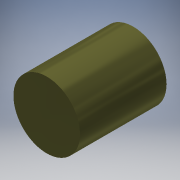
# Autodesk Inventor part: Pin
Saved by Autodesk Inventor 2019 Beta2 (Build 230110000, 110) ContinuousBuild 0
## iProperties
Created: 2014-03-04
Part Number: Pin
Material: Titanium
Document SubType Name: Modeling
Designer: John
Density: 4.51 g/cm^3
Appearance: Titanium
Mass: 1.17905 g
Surface Area: 2.28018 cm^2
Volume: 0.261429 cm^3
Author: John
Autodesk Inventor part; units mm, degrees
ref_plane "YZ Plane" through (0, 0, 0) normal (1, 0, 0) x (0, 1, 0)
ref_plane "XZ Plane" through (0, 0, 0) normal (0, 1, 0) x (-1, 0, 0)
ref_plane "XY Plane" through (0, 0, 0) normal (0, 0, 1) x (1, 0, 0)
sketch "Sketch1" plane through (0, 0, 0) normal (0, 0, 1) x (1, 0, 0)
  circle A0 centre (0, 0) radius 3.175
  dimension "d0" = 6.35
  constraints: 1 centre point, 1 coincident
  measures "d0" diameter of A0
extrude "Extrusion1" add sketch "Sketch1" along normal blind 8.255
body "Solid1"
